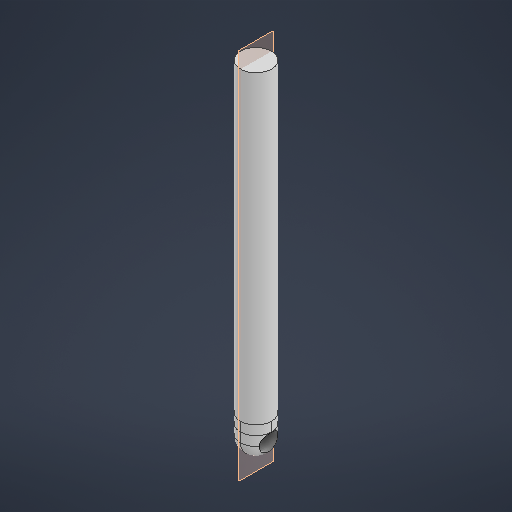
# Autodesk Inventor part: Piston_Bom
Saved by Autodesk Inventor 2026 (Build 300175000, 175)
## iProperties
Created: 2025-05-02
Part Number: Piston_Bom
Material: Generic
Document SubType Name: Modeling
Designer: elias
Density: 1 g/cm^3
Appearance: Default
Author: elias
Autodesk Inventor part; units mm, degrees
ref_plane "XZ Plane" through (0, 0, 0) normal (0, 1, 0) x (-1, 0, 0)
ref_plane "XY Plane" through (0, 0, 0) normal (0, 0, 1) x (1, 0, 0)
sketch "Sketch1" plane through (0, 0, 0) normal (0, 1, 0) x (-1, 0, 0)
  circle A0 centre (0, 0) radius 25
  dimension "d0" = 50
  constraints: 1 centre point, 1 coincident
  measures "d0" diameter of A0
extrude "Extrusion1" add sketch "Sketch1" along normal blind 490
sketch "Sketch2" plane through (0, 0, 0) normal (0, -1, 0) x (1, 0, 0)
  line L0 (-25, -25) -> (25, -25)
  line L1 (25, -25) -> (25, 25)
  line L2 (25, 25) -> (-25, 25)
  line L3 (-25, 25) -> (-25, -25)
  point P0 (0, 0)
  constraints: 8 end point, 2 parallel, 1 horizontal, 1 perpendicular
extrude "Extrusion2" add sketch "Sketch2" along normal blind 60
sketch "Sketch3" plane through (0, 0, 0) normal (1, 0, 0) x (0, 1, 0)
  circle A0 centre (-30, 0) radius 15
  line L0 (0, -25) -> (0, 0) projected
  line L1 (0, 25) -> (-60, 25) projected
  line L2 (0, -25) -> (-60, -25) projected
  arc A1 (-30, 25) -> (-30, -25) centre (-30, 0) ccw
  line L3 (-30, 25) -> (-30, 40.1158)
  line L4 (-30, 40.1158) -> (-76.6193, 40.1158)
  line L5 (-76.6193, 40.1158) -> (-77.4473, -45.6375)
  line L6 (-77.4473, -45.6375) -> (-35.1048, -45.6375)
  line L7 (-35.1048, -45.6375) -> (-30, -25)
  dimension "d5" = 30
  dimension "d6" = 30
  constraints: 10 end point, 2 centre point, 2 midpoint, 2 point on circle, 1 concentric, 1 parallel, 1 perpendicular, 1 vertical
  measures "d5" diameter of A0
  measures "d6" distance from line of L0 A0.centre
extrude "Extrusion3" cut sketch "Sketch3" along normal mid plane 100
fillet "Fillet1" radius 24.9775 6 edges at (25, -55, 0) (25, -15, -25) (25, -15, 25) (-25, -55, 0) (-25, -15, -25) (-25, -15, 25)
body "Solid1"
